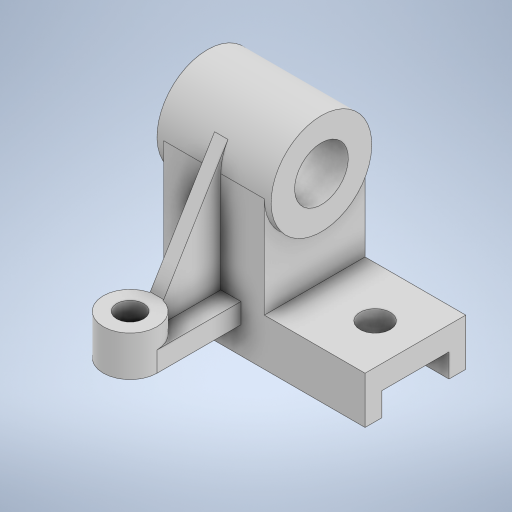
# Autodesk Inventor part: 6
Saved by Autodesk Inventor 2023 (Build 270158000, 158)
## iProperties
Created: 2023-10-17
Part Number: 6
Material: Všeobecné
Document SubType Name: Modeling
Designer: clu40164
Mass: 439.435 g
Surface Area: 628.251 cm^2
Volume: 439.435 cm^3
Density: 1 g/cm^3
Appearance: Výchozí
Author: clu40164
Autodesk Inventor part; units mm, degrees
ref_plane "YZ Plane" through (0, 0, 0) normal (1, 0, 0) x (0, 1, 0)
ref_plane "XZ Plane" through (0, 0, 0) normal (0, 1, 0) x (-1, 0, 0)
ref_plane "XY Plane" through (0, 0, 0) normal (0, 0, 1) x (1, 0, 0)
sketch "Náčrt1" plane through (0, 0, 0) normal (1, 0, 0) x (0, 1, 0)
  circle A0 centre (60, 0) radius 16
  circle A1 centre (60, 0) radius 30
  line L0 (0, 30) -> (0, -30)
  line L1 (0, -30) -> (60, -30)
  line L2 (0, 30) -> (60, 30)
  line L3 (0, 30) -> (0, 68)
  line L4 (0, 68) -> (12, 68)
  line L5 (12, 68) -> (12, 64)
  line L6 (12, 64) -> (75.4986, 25.6864)
  line L7 (0, 68) -> (-12, 68)
  line L8 (-12, 68) -> (-12, 30)
  line L9 (-12, 30) -> (-28, 30)
  line L10 (-28, 30) -> (-28, 20)
  line L11 (-28, 20) -> (-14, 20)
  line L12 (-14, 20) -> (-14, -20)
  line L13 (-14, -20) -> (-28, -20)
  line L14 (-28, -20) -> (-28, -30)
  line L15 (-28, -30) -> (0, -30)
  line L16 (0, 30) -> (-12, 30)
  point P0 (0, 0)
  dimension "d0" = 32
  dimension "d1" = 60
  dimension "d2" = 12
  dimension "d3" = 31.106
  dimension "d4" = 60
  dimension "d5" = 38
  dimension "d6" = 10
  dimension "d7" = 50
  dimension "d8" = 24
  dimension "d9" = 26
  dimension "d10" = 40
  dimension "d11" = 60.9972
  dimension "d12" = 30
  dimension "d13" = 12
  constraints: 34 end point, 10 perpendicular, 3 point on circle, 3 tangent, 2 centre point, 2 horizontal, 2 point on line, 2 vertical, 1 coincident
  measures "d0" diameter of A0
  measures "d1" diameter of A1
  measures "d2" distance of L3.end L4.end
  measures "d3" angle of L2 L6
  measures "d4" distance between parallel lines of L2 L1
  measures "d5" distance between parallel lines of L2 L4
  measures "d6" distance between parallel lines of L2 L11
  measures "d7" distance between parallel lines of L2 L13
  measures "d8" distance between parallel lines of L8 L5
  measures "d9" distance between parallel lines of L5 L12
  measures "d10" distance between parallel lines of L14 L5
  measures "d11" distance from line of point (0, 0) L6
  measures "d12" distance from line of point (0, 0) L2
  measures "d13" distance from line of point (0, 0) L5
extrude "Vysunutí1" add sketch "Náčrt1" against normal blind 34 contours A1
extrude "Vysunutí2" add sketch "Náčrt1" against normal blind 4 contours A1 L2 L3 L4 L5 L6
extrude "Vysunutí3" add sketch "Náčrt1" against normal blind 30 contours L1 L0 L2 A1
extrude "Vysunutí4" add sketch "Náčrt1" against normal blind 16 contours L16 L8 L7 L3
extrude "Vysunutí5" add sketch "Náčrt1" against normal blind 30 contours L15 L14 L13 L12 L11 L10 L9 L16 L0
extrude "Vysunutí6" add sketch "Náčrt1" along normal blind 34 contours A1
extrude "Vysunutí7" add sketch "Náčrt1" along normal blind 30 contours L1 L0 L2 A1
extrude "Vysunutí8" add sketch "Náčrt1" along normal blind 4 contours A1 L2 L3 L4 L5 L6
extrude "Vysunutí9" add sketch "Náčrt1" along normal blind 16 contours L16 L8 L7 L3
extrude "Vysunutí10" add sketch "Náčrt1" along normal blind 90 contours L15 L14 L13 L12 L11 L10 L9 L16 L0
sketch "Náčrt2" plane through (-16, -12, 30) normal (0, -1, 0) x (1, 0, 0)
  circle A0 centre (16, 50) radius 16
  circle A1 centre (16, 50) radius 8
  line L0 (20, 38) -> (32, 38) projected
  line L1 (32, 38) -> (32, 50)
  line L2 (0, 38) -> (0, 50)
  line L3 (32, 38) -> (26.583, 38)
  line L4 (12, 38) -> (0, 38) projected
  line L5 (0, 38) -> (5.417, 38)
  point P0 (16, -30)
  dimension "d34" = 32
  dimension "d35" = 16
  dimension "d36" = 12
  constraints: 8 end point, 4 point on circle, 2 centre point, 2 point on line, 2 tangent, 1 coincident, 1 vertical
  measures "d34" diameter of A0
  measures "d35" diameter of A1
  measures "d36" distance from line of L1.end L4
extrude "Vysunutí11" add sketch "Náčrt2" against normal blind 24 contours A0
extrude "Vysunutí12" add sketch "Náčrt2" against normal blind 12 contours L1 L0 A0 | A0 L4 L2
sketch "Náčrt3" plane through (30, 0, 30) normal (0, 1, 0) x (1, 0, 0)
  circle A0 centre (36, 30) radius 9
  point P0 (-30, 30)
  dimension "d41" = 18
  constraints: 1 centre point
  measures "d41" diameter of A0
extrude "Vysunutí13" cut sketch "Náčrt3" against normal blind 14
